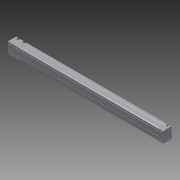
# Autodesk Inventor part: VLA-ST-60-12-0700W Body
Saved by Autodesk Inventor 2011 SP1 (Build 150282100, 282)
## iProperties
Created: 2013-10-23
Part Number: VLA-ST-60-12-0700W Body
Catalog Web Link: www.cadenas.de
Description: with Motor-BW-
Vendor: THK
Document SubType Name: Modeling
Designer: PARTuser1
Manufacturer: THK
Density: 1 g/cm^3
Category: PARTsolutions
Company: THK
Title: VLA-ST-60-12-0700W Body
Author: Cadenas PARTsolutions
PSOL_IDENT_0: {$CADENAS_DATA\23d-libs\thk\actuator\type_vla\slider_type_st\without_motor_1.prj},196 {VTYP=3D},{NB=
PSOL_IDENT_1: VLA-ST-60-12-0700W Body},{LINA=VLA-ST-60-12-0700W Body},{NN=with Motor-BW},{DATE=16.08.2012 09:36:00
PSOL_IDENT_2: },{GEOMDATE=16.08.2012 09:35:00},{VERSION=},{LINEID=230},{LINESUBID=-1},{WBVAR=}  {NB=VLA-ST-60-12-0
PSOL_IDENT_3: 700W Body},{LINA=VLA-ST-60-12-0700W Body},{KT=DUMMY},{IDNR=},{SZ=VLA-ST-60-12-0700},{SZX=60},{ES=700
PSOL_IDENT_4: },{MS=710},{L1=887},{L2=821},{SN=8},{N=9},{M=4.52},{L3=805.000},{NDM=5.000},{P=9.000},{L4=0.000}
CNS_NB: VLA-ST-60-12-0700W Body
CNS_NBSYN: $SZ.W Body
CNS_LINA: VLA-ST-60-12-0700W Body
CNS_SZ: VLA-ST-60-12-0700
CNS_SZX: 60
CNS_ES: 700
CNS_MS: 710
CNS_L1: 887
CNS_L2: 821
CNS_SN: 8
CNS_N: 9
CNS_M: 4.52
CNS_L3: 805.000
CNS_NDM: 5.000
CNS_P: 9.000
CNS_L4: 0.000
SUPPLIER: THK
ARTICLENO: VLA-ST-60-12-0700W Body
BOMINFO: VLA-ST-60-12-0700W Body
CREATOR: CADENAS GmbH
Autodesk Inventor part; units mm, degrees
sketch "Sketch_1" plane through (8, 0, 0) normal (1, 0, 0) x (0, 0, -1)
  line L0 (-32, 45) -> (-32, 30.4)
  line L1 (-32, 30.4) -> (-31, 29.4)
  line L2 (-31, 29.4) -> (-31, 20.4)
  line L3 (-31, 20.4) -> (-32, 19.4)
  line L4 (-32, 19.4) -> (-32, 4.8)
  arc A0 (-32, 4.8) -> (-28, 0.8) centre (-28, 4.8) ccw
  line L5 (-28, 0.8) -> (28, 0.8)
  arc A1 (28, 0.8) -> (32, 4.8) centre (28, 4.8) ccw
  line L6 (32, 4.8) -> (32, 19.4)
  line L7 (32, 19.4) -> (31, 20.4)
  line L8 (31, 20.4) -> (31, 29.4)
  line L9 (31, 29.4) -> (32, 30.4)
  line L10 (32, 30.4) -> (32, 45)
  arc A2 (32, 45) -> (28, 49) centre (28, 45) ccw
  line L11 (28, 49) -> (-28, 49)
  arc A3 (-28, 49) -> (-32, 45) centre (-28, 45) ccw
  line L12 (-31, 44) -> (-31, 30.8142)
  line L13 (-31, 30.8142) -> (-30, 29.8142)
  line L14 (-30, 29.8142) -> (-30, 19.9858)
  line L15 (-30, 19.9858) -> (-31, 18.9858)
  line L16 (-31, 18.9858) -> (-31, 5.8)
  arc A4 (-31, 5.8) -> (-27, 1.8) centre (-27, 5.8) ccw
  line L17 (-27, 1.8) -> (27, 1.8)
  arc A5 (27, 1.8) -> (31, 5.8) centre (27, 5.8) ccw
  line L18 (31, 5.8) -> (31, 18.9858)
  line L19 (31, 18.9858) -> (30, 19.9858)
  line L20 (30, 19.9858) -> (30, 29.8142)
  line L21 (30, 29.8142) -> (31, 30.8142)
  line L22 (31, 30.8142) -> (31, 44)
  arc A6 (31, 44) -> (27, 48) centre (27, 44) ccw
  line L23 (27, 48) -> (-27, 48)
  arc A7 (-27, 48) -> (-31, 44) centre (-27, 44) ccw
  constraints: 48 end point, 16 point on circle, 8 centre point
extrude "Extrusion1" add sketch "Sketch_1" along normal blind 805
sketch "Sketch_2" plane through (8, 0, 0) normal (1, 0, 0) x (0, 0, -1)
  line L0 (-32, 0) -> (32, 0)
  line L1 (32, 0) -> (32, 46.2)
  line L2 (32, 46.2) -> (29.2, 49)
  line L3 (29.2, 49) -> (-29.2, 49)
  line L4 (-29.2, 49) -> (-32, 46.2)
  line L5 (-32, 46.2) -> (-32, 0)
  constraints: 12 end point
extrude "Extrusion2" add sketch "Sketch_2" against normal blind 50
sketch "Sketch_3" plane through (-42, 0, 0) normal (1, 0, 0) x (0, 0, -1)
  line L0 (-32, 0) -> (32, 0)
  line L1 (32, 0) -> (32, 48)
  line L2 (32, 48) -> (28, 52)
  line L3 (28, 52) -> (-28, 52)
  line L4 (-28, 52) -> (-32, 48)
  line L5 (-32, 48) -> (-32, 0)
  constraints: 12 end point
extrude "Extrusion3" add sketch "Sketch_3" against normal blind 10
sketch "Sketch_4" plane through (0, 0, 0) normal (1, 0, 0) x (0, 1, 0)
  line L0 (35, -26) -> (0, -26)
  line L1 (0, -26) -> (0, -23.25)
  line L2 (0, -23.25) -> (35, -23.25)
  line L3 (35, -23.25) -> (35, -26)
  line L4 (35, -26) -> (0, -26)
  constraints: 10 end point
revolve "Revolution1" cut sketch "Sketch_4" angle 360 about axis through (0, 35, -26) along (0, 1, 0)
sketch "Sketch_5" plane through (0, 49, 0) normal (0, 1, 0) x (1, 0, 0)
  arc A0 (-6, 26) -> (6, 26) centre (0, 26) ccw
  line L0 (6, 26) -> (6, 32)
  line L1 (6, 32) -> (-6, 32)
  line L2 (-6, 32) -> (-6, 26)
  constraints: 6 end point, 2 point on circle, 1 centre point
extrude "Extrusion4" cut sketch "Sketch_5" against normal blind 14
sketch "Sketch_6" plane through (0, 0, 0) normal (1, 0, 0) x (0, 1, 0)
  line L0 (35, 26) -> (0, 26)
  line L1 (0, 26) -> (0, 28.75)
  line L2 (0, 28.75) -> (35, 28.75)
  line L3 (35, 28.75) -> (35, 26)
  line L4 (35, 26) -> (0, 26)
  constraints: 10 end point
revolve "Revolution2" cut sketch "Sketch_6" angle 360 about axis through (0, 35, 26) along (0, 1, 0)
sketch "Sketch_7" plane through (0, 49, 0) normal (0, 1, 0) x (1, 0, 0)
  line L0 (-6, -26) -> (-6, -32)
  line L1 (-6, -32) -> (6, -32)
  line L2 (6, -32) -> (6, -26)
  arc A0 (6, -26) -> (-6, -26) centre (0, -26) ccw
  constraints: 6 end point, 2 point on circle, 1 centre point
extrude "Extrusion5" cut sketch "Sketch_7" against normal blind 14
sketch "Sketch_8" plane through (-35, 0, 0) normal (1, 0, 0) x (0, 0, -1)
  line L0 (26, 35) -> (26, 0)
  line L1 (26, 0) -> (23.25, 0)
  line L2 (23.25, 0) -> (23.25, 35)
  line L3 (23.25, 35) -> (26, 35)
  line L4 (26, 35) -> (26, 0)
  constraints: 10 end point
revolve "Revolution3" cut sketch "Sketch_8" angle 360 about axis through (-35, 35, -26) along (0, 1, 0)
sketch "Sketch_9" plane through (-35, 0, 0) normal (1, 0, 0) x (0, 0, -1)
  line L0 (-26, 35) -> (-26, 0)
  line L1 (-26, 0) -> (-28.75, 0)
  line L2 (-28.75, 0) -> (-28.75, 35)
  line L3 (-28.75, 35) -> (-26, 35)
  line L4 (-26, 35) -> (-26, 0)
  constraints: 10 end point
revolve "Revolution4" cut sketch "Sketch_9" angle 360 about axis through (-35, 35, 26) along (0, 1, 0)
sketch "Sketch_10" plane through (0, 49, 0) normal (0, 1, 0) x (1, 0, 0)
  arc A0 (-41, 26) -> (-29, 26) centre (-35, 26) ccw
  line L0 (-29, 26) -> (-29, 32)
  line L1 (-29, 32) -> (-41, 32)
  line L2 (-41, 32) -> (-41, 26)
  constraints: 6 end point, 2 point on circle, 1 centre point
extrude "Extrusion6" cut sketch "Sketch_10" against normal blind 14
sketch "Sketch_11" plane through (0, 49, 0) normal (0, 1, 0) x (1, 0, 0)
  line L0 (-41, -26) -> (-41, -32)
  line L1 (-41, -32) -> (-29, -32)
  line L2 (-29, -32) -> (-29, -26)
  arc A0 (-29, -26) -> (-41, -26) centre (-35, -26) ccw
  constraints: 6 end point, 2 point on circle, 1 centre point
extrude "Extrusion7" cut sketch "Sketch_11" against normal blind 14
sketch "Sketch_12" plane through (812, 0, 0) normal (1, 0, 0) x (0, 0, -1)
  line L0 (-32, 0) -> (32, 0)
  line L1 (32, 0) -> (32, 48)
  line L2 (32, 48) -> (31, 49)
  line L3 (31, 49) -> (-31, 49)
  line L4 (-31, 49) -> (-32, 48)
  line L5 (-32, 48) -> (-32, 0)
  constraints: 12 end point
extrude "Extrusion8" add sketch "Sketch_12" along normal blind 17
sketch "Sketch_13" plane through (829, 0, 0) normal (1, 0, 0) x (0, 0, -1)
  line L0 (-32, 45) -> (-32, 4.8)
  arc A0 (-32, 4.8) -> (-28, 0.8) centre (-28, 4.8) ccw
  line L1 (-28, 0.8) -> (28, 0.8)
  arc A1 (28, 0.8) -> (32, 4.8) centre (28, 4.8) ccw
  line L2 (32, 4.8) -> (32, 45)
  arc A2 (32, 45) -> (28, 49) centre (28, 45) ccw
  line L3 (28, 49) -> (-28, 49)
  arc A3 (-28, 49) -> (-32, 45) centre (-28, 45) ccw
  constraints: 8 end point, 8 point on circle, 4 centre point
extrude "Extrusion9" add sketch "Sketch_13" along normal blind 6
sketch "Sketch_16" plane through (0, 49, 0) normal (0, 1, 0) x (1, 0, 0)
  arc A0 (815, 26) -> (827, 26) centre (821, 26) ccw
  line L0 (827, 26) -> (827, 32)
  line L1 (827, 32) -> (815, 32)
  line L2 (815, 32) -> (815, 26)
  constraints: 6 end point, 2 point on circle, 1 centre point
extrude "Extrusion10" cut sketch "Sketch_16" against normal blind 14
sketch "Sketch_17" plane through (0, 49, 0) normal (0, 1, 0) x (1, 0, 0)
  line L0 (815, -26) -> (815, -32)
  line L1 (815, -32) -> (827, -32)
  line L2 (827, -32) -> (827, -26)
  arc A0 (827, -26) -> (815, -26) centre (821, -26) ccw
  constraints: 6 end point, 2 point on circle, 1 centre point
extrude "Extrusion11" cut sketch "Sketch_17" against normal blind 14
sketch "Sketch_20" plane through (0, 49, 0) normal (0, 1, 0) x (1, 0, 0)
  line L0 (-40, -11) -> (828, -11)
  line L1 (828, -11) -> (828, 11)
  line L2 (828, 11) -> (-40, 11)
  line L3 (-40, 11) -> (-40, -11)
  constraints: 8 end point
extrude "Extrusion12" cut sketch "Sketch_20" against normal blind 0.1
sketch "Sketch_21" plane through (0, 48.7, 0) normal (0, 1, 0) x (1, 0, 0)
  line L0 (-41, -11) -> (-35, -11)
  line L1 (-35, -11) -> (-35, 11)
  line L2 (-35, 11) -> (-41, 11)
  line L3 (-41, 11) -> (-41, -11)
  constraints: 8 end point
sketch "Sketch_22" plane through (0, 48.7, 0) normal (0, 1, 0) x (1, 0, 0)
  line L0 (822, -11) -> (828, -11)
  line L1 (828, -11) -> (828, 11)
  line L2 (828, 11) -> (822, 11)
  line L3 (822, 11) -> (822, -11)
  constraints: 8 end point
sketch "Sketch_14" plane through (0, 35, 0) normal (0, 1, 0) x (1, 0, 0)
  arc A0 (819.75, 28.75) -> (819.75, 23.25) centre (819.9847, 26) ccw
  line L0 (819.75, 23.25) -> (822.25, 23.25)
  arc A1 (822.25, 23.25) -> (822.25, 28.75) centre (822.0153, 26) ccw
  line L1 (822.25, 28.75) -> (819.75, 28.75)
  constraints: 4 end point, 4 point on circle, 2 centre point
extrude "Extrusion13" cut sketch "Sketch_14" against normal blind 35
sketch "Sketch_15" plane through (0, 35, 0) normal (0, 1, 0) x (1, 0, 0)
  arc A0 (819.75, -23.25) -> (819.75, -28.75) centre (819.9847, -26) ccw
  line L0 (819.75, -28.75) -> (822.25, -28.75)
  arc A1 (822.25, -28.75) -> (822.25, -23.25) centre (822.0153, -26) ccw
  line L1 (822.25, -23.25) -> (819.75, -23.25)
  constraints: 4 end point, 4 point on circle, 2 centre point
extrude "Extrusion14" cut sketch "Sketch_15" against normal blind 35
extrude "Extrusion15" add sketch "Sketch_22" along normal blind 0.4
extrude "Extrusion16" add sketch "Sketch_21" along normal blind 0.4
sketch "Sketch_23" plane through (0, 0, 6.5) normal (0, 0, 1) x (1, 0, 0)
  line L0 (-38.01, 49) -> (-38.01, 50)
  line L1 (-38.01, 50) -> (-35.02, 50)
  line L2 (-35.02, 50) -> (-35.02, 49)
  line L3 (-35.02, 49) -> (-38.01, 49)
  line L4 (-38.01, 49) -> (-38.01, 50)
  constraints: 10 end point
revolve "Revolution5" add sketch "Sketch_23" angle 360 about axis through (-38.01, 49, 6.5) along (0, -1, 0)
sketch "Sketch_24" plane through (0, 0, -6.5) normal (0, 0, 1) x (1, 0, 0)
  line L0 (-38.01, 49) -> (-38.01, 50)
  line L1 (-38.01, 50) -> (-35.02, 50)
  line L2 (-35.02, 50) -> (-35.02, 49)
  line L3 (-35.02, 49) -> (-38.01, 49)
  line L4 (-38.01, 49) -> (-38.01, 50)
  constraints: 10 end point
revolve "Revolution6" add sketch "Sketch_24" angle 360 about axis through (-38.01, 49, -6.5) along (0, -1, 0)
sketch "Sketch_25" plane through (0, 0, 6.5) normal (0, 0, 1) x (1, 0, 0)
  line L0 (825, 49) -> (825, 50)
  line L1 (825, 50) -> (827.99, 50)
  line L2 (827.99, 50) -> (827.99, 49)
  line L3 (827.99, 49) -> (825, 49)
  line L4 (825, 49) -> (825, 50)
  constraints: 10 end point
revolve "Revolution7" add sketch "Sketch_25" angle 360 about axis through (825, 49, 6.5) along (0, -1, 0)
sketch "Sketch_26" plane through (0, 0, -6.5) normal (0, 0, 1) x (1, 0, 0)
  line L0 (825, 49) -> (825, 50)
  line L1 (825, 50) -> (827.99, 50)
  line L2 (827.99, 50) -> (827.99, 49)
  line L3 (827.99, 49) -> (825, 49)
  line L4 (825, 49) -> (825, 50)
  constraints: 10 end point
revolve "Revolution8" add sketch "Sketch_26" angle 360 about axis through (825, 49, -6.5) along (0, -1, 0)
sketch "Sketch_27" plane through (11, 0, 0) normal (1, 0, 0) x (0, 0, -1)
  line L0 (32, 25) -> (31, 25)
  line L1 (31, 25) -> (31, 27.99)
  line L2 (31, 27.99) -> (32, 27.99)
  line L3 (32, 27.99) -> (32, 25)
  line L4 (32, 25) -> (31, 25)
  constraints: 10 end point
revolve "Revolution9" add sketch "Sketch_27" angle 360 about axis through (11, 25, -32) along (0, 0, -1)
sketch "Sketch_28" plane through (0, 50, 0) normal (0, 1, 0) x (1, 0, 0)
  line L0 (-39.51, 6.75) -> (-39.51, 6.25)
  line L1 (-39.51, 6.25) -> (-38.26, 6.25)
  line L2 (-38.26, 6.25) -> (-38.26, 5)
  line L3 (-38.26, 5) -> (-37.76, 5)
  line L4 (-37.76, 5) -> (-37.76, 6.25)
  line L5 (-37.76, 6.25) -> (-36.51, 6.25)
  line L6 (-36.51, 6.25) -> (-36.51, 6.75)
  line L7 (-36.51, 6.75) -> (-37.76, 6.75)
  line L8 (-37.76, 6.75) -> (-37.76, 8)
  line L9 (-37.76, 8) -> (-38.26, 8)
  line L10 (-38.26, 8) -> (-38.26, 6.75)
  line L11 (-38.26, 6.75) -> (-39.51, 6.75)
  constraints: 24 end point
extrude "Extrusion17" cut sketch "Sketch_28" against normal blind 0.5
sketch "Sketch_29" plane through (0, 50, 0) normal (0, 1, 0) x (1, 0, 0)
  line L0 (-39.51, -6.25) -> (-39.51, -6.75)
  line L1 (-39.51, -6.75) -> (-38.26, -6.75)
  line L2 (-38.26, -6.75) -> (-38.26, -8)
  line L3 (-38.26, -8) -> (-37.76, -8)
  line L4 (-37.76, -8) -> (-37.76, -6.75)
  line L5 (-37.76, -6.75) -> (-36.51, -6.75)
  line L6 (-36.51, -6.75) -> (-36.51, -6.25)
  line L7 (-36.51, -6.25) -> (-37.76, -6.25)
  line L8 (-37.76, -6.25) -> (-37.76, -5)
  line L9 (-37.76, -5) -> (-38.26, -5)
  line L10 (-38.26, -5) -> (-38.26, -6.25)
  line L11 (-38.26, -6.25) -> (-39.51, -6.25)
  constraints: 24 end point
extrude "Extrusion18" cut sketch "Sketch_29" against normal blind 0.5
sketch "Sketch_30" plane through (0, 50, 0) normal (0, 1, 0) x (1, 0, 0)
  line L0 (823.5, 6.75) -> (823.5, 6.25)
  line L1 (823.5, 6.25) -> (824.75, 6.25)
  line L2 (824.75, 6.25) -> (824.75, 5)
  line L3 (824.75, 5) -> (825.25, 5)
  line L4 (825.25, 5) -> (825.25, 6.25)
  line L5 (825.25, 6.25) -> (826.5, 6.25)
  line L6 (826.5, 6.25) -> (826.5, 6.75)
  line L7 (826.5, 6.75) -> (825.25, 6.75)
  line L8 (825.25, 6.75) -> (825.25, 8)
  line L9 (825.25, 8) -> (824.75, 8)
  line L10 (824.75, 8) -> (824.75, 6.75)
  line L11 (824.75, 6.75) -> (823.5, 6.75)
  constraints: 24 end point
extrude "Extrusion19" cut sketch "Sketch_30" against normal blind 0.5
sketch "Sketch_31" plane through (0, 50, 0) normal (0, 1, 0) x (1, 0, 0)
  line L0 (823.5, -6.25) -> (823.5, -6.75)
  line L1 (823.5, -6.75) -> (824.75, -6.75)
  line L2 (824.75, -6.75) -> (824.75, -8)
  line L3 (824.75, -8) -> (825.25, -8)
  line L4 (825.25, -8) -> (825.25, -6.75)
  line L5 (825.25, -6.75) -> (826.5, -6.75)
  line L6 (826.5, -6.75) -> (826.5, -6.25)
  line L7 (826.5, -6.25) -> (825.25, -6.25)
  line L8 (825.25, -6.25) -> (825.25, -5)
  line L9 (825.25, -5) -> (824.75, -5)
  line L10 (824.75, -5) -> (824.75, -6.25)
  line L11 (824.75, -6.25) -> (823.5, -6.25)
  constraints: 24 end point
extrude "Extrusion20" cut sketch "Sketch_31" against normal blind 0.5
sketch "Sketch_32" plane through (808, 0, 0) normal (1, 0, 0) x (0, 0, -1)
  line L0 (32, 25) -> (31, 25)
  line L1 (31, 25) -> (31, 27.99)
  line L2 (31, 27.99) -> (32, 27.99)
  line L3 (32, 27.99) -> (32, 25)
  line L4 (32, 25) -> (31, 25)
  constraints: 10 end point
revolve "Revolution10" add sketch "Sketch_32" angle 360 about axis through (808, 25, -32) along (0, 0, -1)
sketch "Sketch_33" plane through (808, 0, 0) normal (1, 0, 0) x (0, 0, -1)
  line L0 (-31, 25) -> (-32, 25)
  line L1 (-32, 25) -> (-32, 27.99)
  line L2 (-32, 27.99) -> (-31, 27.99)
  line L3 (-31, 27.99) -> (-31, 25)
  line L4 (-31, 25) -> (-32, 25)
  constraints: 10 end point
revolve "Revolution11" add sketch "Sketch_33" angle 360 about axis through (808, 25, 31) along (0, 0, -1)
sketch "Sketch_34" plane through (11, 0, 0) normal (1, 0, 0) x (0, 0, -1)
  line L0 (-31, 25) -> (-32, 25)
  line L1 (-32, 25) -> (-32, 27.99)
  line L2 (-32, 27.99) -> (-31, 27.99)
  line L3 (-31, 27.99) -> (-31, 25)
  line L4 (-31, 25) -> (-32, 25)
  constraints: 10 end point
revolve "Revolution12" add sketch "Sketch_34" angle 360 about axis through (11, 25, 31) along (0, 0, -1)
sketch "Sketch_35" plane through (0, 0, 32) normal (0, 0, 1) x (1, 0, 0)
  line L0 (9.5, 25.25) -> (9.5, 24.75)
  line L1 (9.5, 24.75) -> (10.75, 24.75)
  line L2 (10.75, 24.75) -> (10.75, 23.5)
  line L3 (10.75, 23.5) -> (11.25, 23.5)
  line L4 (11.25, 23.5) -> (11.25, 24.75)
  line L5 (11.25, 24.75) -> (12.5, 24.75)
  line L6 (12.5, 24.75) -> (12.5, 25.25)
  line L7 (12.5, 25.25) -> (11.25, 25.25)
  line L8 (11.25, 25.25) -> (11.25, 26.5)
  line L9 (11.25, 26.5) -> (10.75, 26.5)
  line L10 (10.75, 26.5) -> (10.75, 25.25)
  line L11 (10.75, 25.25) -> (9.5, 25.25)
  constraints: 24 end point
extrude "Extrusion21" cut sketch "Sketch_35" against normal blind 0.5
sketch "Sketch_36" plane through (0, 0, 32) normal (0, 0, 1) x (1, 0, 0)
  line L0 (806.5, 25.25) -> (806.5, 24.75)
  line L1 (806.5, 24.75) -> (807.75, 24.75)
  line L2 (807.75, 24.75) -> (807.75, 23.5)
  line L3 (807.75, 23.5) -> (808.25, 23.5)
  line L4 (808.25, 23.5) -> (808.25, 24.75)
  line L5 (808.25, 24.75) -> (809.5, 24.75)
  line L6 (809.5, 24.75) -> (809.5, 25.25)
  line L7 (809.5, 25.25) -> (808.25, 25.25)
  line L8 (808.25, 25.25) -> (808.25, 26.5)
  line L9 (808.25, 26.5) -> (807.75, 26.5)
  line L10 (807.75, 26.5) -> (807.75, 25.25)
  line L11 (807.75, 25.25) -> (806.5, 25.25)
  constraints: 24 end point
extrude "Extrusion22" cut sketch "Sketch_36" against normal blind 0.5
sketch "Sketch_37" plane through (0, 0, -32) normal (0, 0, 1) x (1, 0, 0)
  line L0 (9.5, 25.25) -> (9.5, 24.75)
  line L1 (9.5, 24.75) -> (10.75, 24.75)
  line L2 (10.75, 24.75) -> (10.75, 23.5)
  line L3 (10.75, 23.5) -> (11.25, 23.5)
  line L4 (11.25, 23.5) -> (11.25, 24.75)
  line L5 (11.25, 24.75) -> (12.5, 24.75)
  line L6 (12.5, 24.75) -> (12.5, 25.25)
  line L7 (12.5, 25.25) -> (11.25, 25.25)
  line L8 (11.25, 25.25) -> (11.25, 26.5)
  line L9 (11.25, 26.5) -> (10.75, 26.5)
  line L10 (10.75, 26.5) -> (10.75, 25.25)
  line L11 (10.75, 25.25) -> (9.5, 25.25)
  constraints: 24 end point
extrude "Extrusion23" cut sketch "Sketch_37" along normal blind 0.5
sketch "Sketch_38" plane through (0, 0, -32) normal (0, 0, 1) x (1, 0, 0)
  line L0 (806.5, 25.25) -> (806.5, 24.75)
  line L1 (806.5, 24.75) -> (807.75, 24.75)
  line L2 (807.75, 24.75) -> (807.75, 23.5)
  line L3 (807.75, 23.5) -> (808.25, 23.5)
  line L4 (808.25, 23.5) -> (808.25, 24.75)
  line L5 (808.25, 24.75) -> (809.5, 24.75)
  line L6 (809.5, 24.75) -> (809.5, 25.25)
  line L7 (809.5, 25.25) -> (808.25, 25.25)
  line L8 (808.25, 25.25) -> (808.25, 26.5)
  line L9 (808.25, 26.5) -> (807.75, 26.5)
  line L10 (807.75, 26.5) -> (807.75, 25.25)
  line L11 (807.75, 25.25) -> (806.5, 25.25)
  constraints: 24 end point
extrude "Extrusion24" cut sketch "Sketch_38" along normal blind 0.5
sketch "Sketch37" plane through (835, 0, 0) normal (1, 0, 0) x (0, 0, -1)
  point P0 (18, 32)
hole "Drilling 5" at (835, 32, -18) direction (-1, 0, 0) diameter 7 depth 2
sketch "Sketch38" plane through (835, 0, 0) normal (1, 0, 0) x (0, 0, -1)
  point P0 (-18, 32)
hole "Drilling 6" at (835, 32, 18) direction (-1, 0, 0) diameter 7 depth 2
sketch "Sketch_41" plane through (0, 0, 18) normal (0, 0, 1) x (1, 0, 0)
  line L0 (835, 32) -> (833, 32)
  line L1 (833, 32) -> (833, 35)
  line L2 (833, 35) -> (834, 35)
  arc A0 (835, 32) -> (834, 35) centre (830.5031, 32.1677) ccw
  line L3 (835, 32) -> (833, 32)
  constraints: 8 end point, 2 point on circle, 1 centre point
revolve "Revolution13" add sketch "Sketch_41" angle 360 about axis through (835, 32, 18) along (1, 0, 0)
sketch "Sketch_42" plane through (835, 0, 0) normal (1, 0, 0) x (0, 0, -1)
  line L0 (-19.2374, 32.8839) -> (-18.3536, 32)
  line L1 (-18.3536, 32) -> (-19.2374, 31.1161)
  line L2 (-19.2374, 31.1161) -> (-18.8839, 30.7626)
  line L3 (-18.8839, 30.7626) -> (-18, 31.6464)
  line L4 (-18, 31.6464) -> (-17.1161, 30.7626)
  line L5 (-17.1161, 30.7626) -> (-16.7626, 31.1161)
  line L6 (-16.7626, 31.1161) -> (-17.6464, 32)
  line L7 (-17.6464, 32) -> (-16.7626, 32.8839)
  line L8 (-16.7626, 32.8839) -> (-17.1161, 33.2374)
  line L9 (-17.1161, 33.2374) -> (-18, 32.3536)
  line L10 (-18, 32.3536) -> (-18.8839, 33.2374)
  line L11 (-18.8839, 33.2374) -> (-19.2374, 32.8839)
  constraints: 24 end point
extrude "Extrusion25" cut sketch "Sketch_42" along normal mid plane 1.6
sketch "Sketch_43" plane through (835, 0, 0) normal (1, 0, 0) x (0, 0, -1)
  line L0 (16.7626, 32.8839) -> (17.6464, 32)
  line L1 (17.6464, 32) -> (16.7626, 31.1161)
  line L2 (16.7626, 31.1161) -> (17.1161, 30.7626)
  line L3 (17.1161, 30.7626) -> (18, 31.6464)
  line L4 (18, 31.6464) -> (18.8839, 30.7626)
  line L5 (18.8839, 30.7626) -> (19.2374, 31.1161)
  line L6 (19.2374, 31.1161) -> (18.3536, 32)
  line L7 (18.3536, 32) -> (19.2374, 32.8839)
  line L8 (19.2374, 32.8839) -> (18.8839, 33.2374)
  line L9 (18.8839, 33.2374) -> (18, 32.3536)
  line L10 (18, 32.3536) -> (17.1161, 33.2374)
  line L11 (17.1161, 33.2374) -> (16.7626, 32.8839)
  constraints: 24 end point
sketch "Sketch_44" plane through (0, 0, -18) normal (0, 0, 1) x (1, 0, 0)
  line L0 (835, 32) -> (833, 32)
  line L1 (833, 32) -> (833, 35)
  line L2 (833, 35) -> (834, 35)
  arc A0 (835, 32) -> (834, 35) centre (830.5031, 32.1677) ccw
  line L3 (835, 32) -> (833, 32)
  constraints: 8 end point, 2 point on circle, 1 centre point
revolve "Revolution14" add sketch "Sketch_44" angle 360 about axis through (835, 32, -18) along (1, 0, 0)
extrude "Extrusion26" cut sketch "Sketch_43" along normal mid plane 1.6
sketch "Sketch_56" plane through (0, 0, 16.2635) normal (0, 0, 1) x (1, 0, 0)
  line L0 (-47, 15.7365) -> (-52, 15.7365)
  line L1 (-52, 15.7365) -> (-52, 17.7365)
  line L2 (-52, 17.7365) -> (-51.621, 17.3575)
  line L3 (-51.621, 17.3575) -> (-48.379, 17.3575)
  line L4 (-48.379, 17.3575) -> (-48, 17.7365)
  line L5 (-48, 17.7365) -> (-47, 15.7365)
  line L6 (-47, 15.7365) -> (-52, 15.7365)
  constraints: 14 end point
revolve "Revolution15" cut sketch "Sketch_56" angle 360 about axis through (-47, 15.7365, 16.2635) along (1, 0, 0)
thread "Thread1" size "M4x0.7" class "6H" standard "ISO Metric profile" full length
sketch "Sketch_57" plane through (0, 0, 16.2635) normal (0, 0, 1) x (1, 0, 0)
  line L0 (-47, 48.2635) -> (-52, 48.2635)
  line L1 (-52, 48.2635) -> (-52, 50.2635)
  line L2 (-52, 50.2635) -> (-51.621, 49.8845)
  line L3 (-51.621, 49.8845) -> (-48.379, 49.8845)
  line L4 (-48.379, 49.8845) -> (-48, 50.2635)
  line L5 (-48, 50.2635) -> (-47, 48.2635)
  line L6 (-47, 48.2635) -> (-52, 48.2635)
  constraints: 14 end point
revolve "Revolution16" cut sketch "Sketch_57" angle 360 about axis through (-47, 48.2635, 16.2635) along (1, 0, 0)
thread "Thread2" size "M4x0.7" class "6H" standard "ISO Metric profile" full length
sketch "Sketch_62" plane through (0, 0, -16.2635) normal (0, 0, 1) x (1, 0, 0)
  line L0 (-47, 15.7365) -> (-52, 15.7365)
  line L1 (-52, 15.7365) -> (-52, 17.7365)
  line L2 (-52, 17.7365) -> (-51.621, 17.3575)
  line L3 (-51.621, 17.3575) -> (-48.379, 17.3575)
  line L4 (-48.379, 17.3575) -> (-48, 17.7365)
  line L5 (-48, 17.7365) -> (-47, 15.7365)
  line L6 (-47, 15.7365) -> (-52, 15.7365)
  constraints: 14 end point
revolve "Revolution17" cut sketch "Sketch_62" angle 360 about axis through (-47, 15.7365, -16.2635) along (1, 0, 0)
thread "Thread3" size "M4x0.7" class "6H" standard "ISO Metric profile" full length
sketch "Sketch_61" plane through (0, 0, -16.2635) normal (0, 0, 1) x (1, 0, 0)
  line L0 (-47, 48.2635) -> (-52, 48.2635)
  line L1 (-52, 48.2635) -> (-52, 50.2635)
  line L2 (-52, 50.2635) -> (-51.621, 49.8845)
  line L3 (-51.621, 49.8845) -> (-48.379, 49.8845)
  line L4 (-48.379, 49.8845) -> (-48, 50.2635)
  line L5 (-48, 50.2635) -> (-47, 48.2635)
  line L6 (-47, 48.2635) -> (-52, 48.2635)
  constraints: 14 end point
revolve "Revolution18" cut sketch "Sketch_61" angle 360 about axis through (-47, 48.2635, -16.2635) along (1, 0, 0)
thread "Thread4" size "M4x0.7" class "6H" standard "ISO Metric profile" full length
sketch "Sketch47" plane through (-52, 0, 0) normal (-1, 0, 0) x (0, 0, 1)
  point P0 (0, 32)
hole "Drilling 7" at (-52, 32, 0) direction (1, 0, 0) diameter 30 depth 3
sketch "Sketch_46" plane through (-50, 0, 0) normal (1, 0, 0) x (0, 0, -1)
  circle A0 centre (0, 32) radius 14
  constraints: 1 centre point
extrude "Extrusion27" cut sketch "Sketch_46" along normal blind 41
sketch "Sketch_47" plane through (-9, 0, 0) normal (1, 0, 0) x (0, 0, -1)
  arc A0 (-7.4246, 33.0607) -> (-7.4246, 30.9393) centre (0, 32) ccw
  line L0 (-7.4246, 30.9393) -> (-1.0607, 24.5754)
  arc A1 (-1.0607, 24.5754) -> (1.0607, 24.5754) centre (0, 32) ccw
  line L1 (1.0607, 24.5754) -> (7.4246, 30.9393)
  arc A2 (7.4246, 30.9393) -> (7.4246, 33.0607) centre (0, 32) ccw
  line L2 (7.4246, 33.0607) -> (1.0607, 39.4246)
  arc A3 (1.0607, 39.4246) -> (-1.0607, 39.4246) centre (0, 32) ccw
  line L3 (-1.0607, 39.4246) -> (-7.4246, 33.0607)
  constraints: 8 end point, 8 point on circle, 4 centre point
extrude "Extrusion28" add sketch "Sketch_47" against normal blind 6
sketch "Sketch_48" plane through (-9, 0, 0) normal (1, 0, 0) x (0, 0, -1)
  circle A0 centre (0, 32) radius 6.95
  constraints: 1 centre point
extrude "Extrusion29" cut sketch "Sketch_48" along normal blind 3
sketch "Sketch_49" plane through (0, 0, 0) normal (0, 0, 1) x (1, 0, 0)
  line L0 (-15, 32) -> (-23, 32)
  line L1 (-23, 32) -> (-23, 34.2)
  line L2 (-23, 34.2) -> (-22.2, 35)
  line L3 (-22.2, 35) -> (-15, 35)
  line L4 (-15, 35) -> (-15, 32)
  line L5 (-15, 32) -> (-23, 32)
  constraints: 12 end point
revolve "Revolution19" add sketch "Sketch_49" angle 360 about axis through (-15, 32, 0) along (1, 0, 0)
sketch "Sketch_50" plane through (0, 0, 0) normal (0, 0, 1) x (1, 0, 0)
  line L0 (814, 32) -> (7, 32)
  line L1 (7, 32) -> (7, 35.5)
  line L2 (7, 35.5) -> (814, 35.5)
  line L3 (814, 35.5) -> (814, 32)
  line L4 (814, 32) -> (7, 32)
  constraints: 10 end point
revolve "Revolution20" add sketch "Sketch_50" angle 360 about axis through (814, 32, 0) along (1, 0, 0)
sketch "Sketch_51" plane through (-52, 0, 0) normal (1, 0, 0) x (0, 0, -1)
  line L0 (-21, 0) -> (21, 0)
  line L1 (21, 0) -> (21, 9)
  line L2 (21, 9) -> (-21, 9)
  line L3 (-21, 9) -> (-21, 0)
  constraints: 8 end point
extrude "Extrusion30" cut sketch "Sketch_51" along normal blind 882
sketch "Sketch_52" plane through (-52, 0, 0) normal (1, 0, 0) x (0, 0, -1)
  line L0 (-21, 2.1) -> (-21, 0.5)
  line L1 (-21, 0.5) -> (-20.5, 0)
  line L2 (-20.5, 0) -> (-8, 0)
  line L3 (-8, 0) -> (-7.7, 0.3)
  line L4 (-7.7, 0.3) -> (8, 0.3)
  line L5 (8, 0.3) -> (8.3, 0)
  line L6 (8.3, 0) -> (20.5, 0)
  line L7 (20.5, 0) -> (21, 0.5)
  line L8 (21, 0.5) -> (21, 2.1)
  line L9 (21, 2.1) -> (20, 3.1)
  line L10 (20, 3.1) -> (20, 5.3)
  arc A0 (20, 8.3) -> (20, 5.3) centre (20.9014, 6.8) ccw
  line L11 (20, 8.3) -> (20, 8.7)
  line L12 (20, 8.7) -> (19.7, 9)
  line L13 (19.7, 9) -> (-19.7, 9)
  line L14 (-19.7, 9) -> (-20, 8.7)
  line L15 (-20, 8.7) -> (-20, 8.3)
  arc A1 (-20, 5.3) -> (-20, 8.3) centre (-20.9014, 6.8) ccw
  line L16 (-20, 5.3) -> (-20, 3.1)
  line L17 (-20, 3.1) -> (-21, 2.1)
  constraints: 36 end point, 4 point on circle, 2 centre point
extrude "Extrusion31" add sketch "Sketch_52" along normal blind 881
sketch "Sketch55" plane through (-52, 0, -8.3) normal (0, -1, 0) x (1, 0, 0)
  point P0 (840, -4.2)
hole "Drilling 10" at (788, 0, -12.5) direction (0, 1, 0) diameter 4.134 depth 9 countersink diameter 5 countersink angle 90 thread size "M5x0.8" class "6H" standard "ISO Metric profile"
sketch "Sketch56" plane through (-52, 0, 20.5) normal (0, -1, 0) x (1, 0, 0)
  point P0 (840, -8)
hole "Drilling 11" at (788, 0, 12.5) direction (0, 1, 0) diameter 4.134 depth 9 countersink diameter 5 countersink angle 90 thread size "M5x0.8" class "6H" standard "ISO Metric profile"
pattern_linear "Rectangular Pattern1" count 9 spacing 100 along (-1, 0, 0) of "Drilling 11"
pattern_linear "Rectangular Pattern2" count 9 spacing 100 along (-1, 0, 0) of "Drilling 10"
sketch "Sketch_18" plane through (0, 0, 0) normal (1, 0, 0) x (0, 1, 0)
  line L0 (30, 27.5) -> (30, 32)
  line L1 (30, 32) -> (31.3, 32)
  line L2 (31.3, 32) -> (31.3, 27.5)
  line L3 (31.3, 27.5) -> (30, 27.5)
  line L4 (30, 27.5) -> (30, 32)
  constraints: 10 end point
revolve "Revolution21" cut sketch "Sketch_18" angle 360 about axis through (0, 30, 27.5) along (0, 0, -1)
sketch "Sketch58" plane through (8, 0, -32) normal (0, 0, -1) x (-1, 0, 0)
  point P0 (8, 30)
hole "Drilling 13" at (0, 30, -32) direction (0, 0, 1) diameter 2.6 depth 4.5
sketch "Sketch_63" plane through (821, 0, 0) normal (1, 0, 0) x (0, 0, -1)
  line L0 (-27.5, 30) -> (-32, 30)
  line L1 (-32, 30) -> (-32, 31.3)
  line L2 (-32, 31.3) -> (-27.5, 31.3)
  line L3 (-27.5, 31.3) -> (-27.5, 30)
  line L4 (-27.5, 30) -> (-32, 30)
  constraints: 10 end point
revolve "Revolution22" cut sketch "Sketch_63" angle 360 about axis through (821, 30, 27.5) along (0, 0, -1)
sketch "Sketch60" plane through (8, 0, -32) normal (0, 0, -1) x (-1, 0, 0)
  point P0 (-813, 30)
hole "Drilling 15" at (821, 30, -32) direction (0, 0, 1) diameter 2.6 depth 4.5
ref_plane "without_motor_b1_XY" through (0, 0, 0) normal (0, 1, 0) x (1, 0, 0)
ref_plane "without_motor_b1_YZ" through (0, 0, 0) normal (1, 0, 0) x (0, 0, -1)
ref_plane "without_motor_b1_ZX" through (0, 0, 0) normal (0, 0, -1) x (0, 1, 0)
ref_plane "without_motor_b2_XY" through (53.5, 32, 0) normal (-1, 0, 0) x (0, 0, -1)
ref_plane "without_motor_b2_YZ" through (53.5, 32, 0) normal (0, 0, -1) x (0, -1, 0)
ref_plane "without_motor_b2_ZX" through (53.5, 32, 0) normal (0, -1, 0) x (-1, 0, 0)
body "Solid1"
